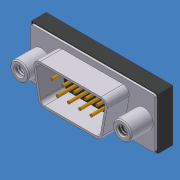
# Autodesk Inventor part: cRIO-FRC 9M D-Shell
Saved by Autodesk Inventor 2011 (Build 150239000, 239)
## iProperties
Category: FRC Parts
Manager: Ed Sparks
Company: FirstCadLibrary
Shininess: 64.0
Length Units: 11269
Angle Units: 11279
Time Units: 11290
Mass Units: 11283
Length Display Precision: 3
Angle Display Precision: 2
Compacted: True
Part Number: cRIO-FRC 9M D-Shell
Document SubType Name: Modeling
Created: 2005-12-27
Material: ABS Plastic
Designer: Ed Sparks
Project: FIRST
Density: 1 g/cm^3
Density: 0.0
Volumn: 0.0
Area: 0.0
PropertySet Name: Model Information
Control State: 0
Master: False
Checked Out: False
Author: Ed Sparks
Keywords: FIRST
Autodesk Inventor part; units mm, degrees
ref_plane "YZ Plane" through (0, 0, 0) normal (1, 0, 0) x (0, 1, 0)
ref_plane "XZ Plane" through (0, 0, 0) normal (0, 1, 0) x (-1, 0, 0)
ref_plane "XY Plane" through (0, 0, 0) normal (0, 0, 1) x (1, 0, 0)
sketch "Sketch1" plane through (0, 0, 0) normal (0, 0, 1) x (1, 0, 0)
  line L0 (-15.405, 0) -> (15.405, 0)
  line L1 (15.405, 0) -> (15.405, 3.6)
  line L2 (15.405, 3.6) -> (8.48, 3.6)
  line L3 (8.48, 3.6) -> (8.48, 9.96)
  line L4 (8.48, 9.96) -> (-8.48, 9.96)
  line L5 (-8.48, 9.96) -> (-8.48, 3.6)
  line L6 (-8.48, 3.6) -> (-15.405, 3.6)
  line L7 (-15.405, 3.6) -> (-15.405, 0)
  point P0 (0, 0)
  point P1 (0, 0)
  dimension "d0" = 16.96
  dimension "d1" = 9.96
  dimension "d2" = 3.6
  dimension "d3" = 30.81
  constraints: 16 end point, 6 parallel, 3 equal length, 1 coincident, 1 horizontal, 1 midpoint, 1 perpendicular, 1 other
  measures "d0" distance of L3.end L4.end
  measures "d1" distance between parallel lines of L0 L4
  measures "d2" distance of L0.end L1.end
  measures "d3" distance of L0.start L0.end
extrude "Extrusion1" add sketch "Sketch1" along normal blind 0.0001
sketch "Sketch2" plane through (0, 0, 0) normal (0, 0, -1) x (-1, 0, 0)
  line L0 (15.405, 3.6) -> (15.405, 0) projected
  line L1 (-15.405, 0) -> (15.405, 0)
  line L2 (15.405, 0) -> (15.405, 12.58)
  line L3 (15.405, 12.58) -> (-15.405, 12.58)
  line L4 (-15.405, 12.58) -> (-15.405, 0)
  dimension "d6" = 12.58
  constraints: 8 end point, 2 parallel, 1 collinear, 1 horizontal, 1 perpendicular
  measures "d6" distance of L3.end L1.start
extrude "Extrusion2" add sketch "Sketch2" along normal blind 3.6
sketch "Sketch5" plane through (0, 0, -3.6) normal (0, 0, -1) x (-1, 0, 0)
  line L0 (15.405, 0) -> (-15.405, 0) projected
  line L1 (-15.405, 12.58) -> (15.405, 12.58) projected
  line L2 (-7.4102, 10.415) -> (7.4102, 10.415)
  line L3 (8.395, 9.2414) -> (7.293, 2.9914)
  line L4 (6.3081, 2.165) -> (-6.3081, 2.165)
  line L5 (-7.293, 2.9914) -> (-8.395, 9.2414)
  arc A0 (-7.4102, 10.415) -> (-8.395, 9.2414) centre (-7.4102, 9.415) ccw
  arc A1 (8.395, 9.2414) -> (7.4102, 10.415) centre (7.4102, 9.415) ccw
  arc A2 (-7.293, 2.9914) -> (-6.3081, 2.165) centre (-6.3081, 3.165) ccw
  arc A3 (6.3081, 2.165) -> (7.293, 2.9914) centre (6.3081, 3.165) ccw
  line L6 (0, 12.58) -> (0, 0) construction
  line L7 (0, 10.415) -> (0, 12.58) construction
  line L8 (0, 0) -> (0, 2.165) construction
  arc A4 (-7.4102, 10.915) -> (-8.8874, 9.1545) centre (-7.4102, 9.415) ccw
  line L9 (-7.4102, 10.915) -> (7.4102, 10.915)
  arc A5 (8.8874, 9.1545) -> (7.4102, 10.915) centre (7.4102, 9.415) ccw
  line L10 (8.8874, 9.1545) -> (7.7854, 2.9045)
  arc A6 (6.3081, 1.665) -> (7.7854, 2.9045) centre (6.3081, 3.165) ccw
  line L11 (6.3081, 1.665) -> (-6.3081, 1.665)
  arc A7 (-7.7854, 2.9045) -> (-6.3081, 1.665) centre (-6.3081, 3.165) ccw
  line L12 (-7.7854, 2.9045) -> (-8.8874, 9.1545)
  dimension "d22" = 100
  dimension "d23" = 100
  dimension "d24" = 1
  dimension "d25" = 1
  dimension "d26" = 8.25
  dimension "d27" = 16.79
  dimension "d29" = 0.5
  constraints: 22 end point, 16 point on circle, 8 centre point, 8 tangent, 4 midpoint, 3 parallel, 2 collinear, 2 equal radius, 2 point on line, 7 other
  measures "d22" angle of L5 L4
  measures "d23" angle of L3 L4
  measures "d24" radius of A0
  measures "d25" radius of A2
  measures "d26" distance between parallel lines of L4 L2
  measures "d27" distance of L3.start L5.end
  measures "d29" distance between parallel lines of L11 L4
extrude "Extrusion3" add sketch "Sketch5" along normal blind 5.9
sketch "Sketch6" plane through (0, 0, -3.6) normal (0, 0, -1) x (-1, 0, 0)
  line L0 (-15.405, 0) -> (-15.405, 12.58) projected
  line L1 (15.405, 0) -> (-15.405, 0) projected
  line L2 (15.405, 12.58) -> (15.405, 0) projected
  line L3 (-15.405, 12.58) -> (15.405, 12.58) projected
  line L4 (-7.4102, 10.915) -> (7.4102, 10.915) projected
  arc A0 (8.8874, 9.1545) -> (7.4102, 10.915) centre (7.4102, 9.415) ccw projected
  line L5 (8.8874, 9.1545) -> (7.7854, 2.9045) projected
  arc A1 (6.3081, 1.665) -> (7.7854, 2.9045) centre (6.3081, 3.165) ccw projected
  line L6 (6.3081, 1.665) -> (-6.3081, 1.665) projected
  arc A2 (-7.7854, 2.9045) -> (-6.3081, 1.665) centre (-6.3081, 3.165) ccw projected
  line L7 (-7.7854, 2.9045) -> (-8.8874, 9.1545) projected
  arc A3 (-7.4102, 10.915) -> (-8.8874, 9.1545) centre (-7.4102, 9.415) ccw projected
  line L8 (-15.155, 11.83) -> (-15.155, 0.75)
  line L9 (-14.655, 0.25) -> (14.655, 0.25)
  line L10 (15.155, 0.75) -> (15.155, 11.83)
  line L11 (14.655, 12.33) -> (-14.655, 12.33)
  line L12 (-8.395, 9.2414) -> (-7.293, 2.9914) projected
  arc A4 (-7.293, 2.9914) -> (-6.3081, 2.165) centre (-6.3081, 3.165) ccw projected
  line L13 (-6.3081, 2.165) -> (6.3081, 2.165) projected
  arc A5 (-14.655, 12.33) -> (-15.155, 11.83) centre (-14.655, 11.83) ccw
  arc A6 (15.155, 11.83) -> (14.655, 12.33) centre (14.655, 11.83) ccw
  arc A7 (14.655, 0.25) -> (15.155, 0.75) centre (14.655, 0.75) ccw
  arc A8 (-15.155, 0.75) -> (-14.655, 0.25) centre (-14.655, 0.75) ccw
  dimension "d32" = 0.25
  dimension "d33" = 0.5
  constraints: 8 end point, 8 point on circle, 8 tangent, 4 centre point, 3 equal radius, 3 other
  measures "d32" distance between parallel lines of L8 L0
  measures "d33" radius of A5
extrude "Extrusion4" add sketch "Sketch6" along normal blind 0.5 contours A5 L11 A6 L10 A7 L9 A8 L8
sketch "Sketch7" plane through (0, 0, -4.1) normal (0, 0, -1) x (-1, 0, 0)
  line L0 (-14.655, 12.33) -> (14.655, 12.33) projected
  line L1 (14.655, 0.25) -> (-14.655, 0.25) projected
  circle A0 centre (12.495, 6.29) radius 2.25
  line L2 (12.495, 6.29) -> (12.495, 12.33)
  line L3 (12.495, 6.29) -> (12.495, 0.25)
  line L4 (15.405, 12.58) -> (15.405, 0) projected
  dimension "d36" = 4.5
  dimension "d37" = 2.91
  constraints: 4 end point, 2 perpendicular, 2 point on line, 1 centre point, 1 collinear
  measures "d36" diameter of A0
  measures "d37" distance from line of L4 L2.start
extrude "Extrusion5" add sketch "Sketch7" along normal blind 5.4
sketch "Sketch8" plane through (-12.495, 6.29, -9.5) normal (0, 0, -1) x (-1, 0, 0)
  circle A0 centre (0, 0) radius 2.25 projected
  constraints: 1 coincident
hole "Hole2" at (-12.495, 6.29, -9.5) direction (0, 0, 1) diameter 2.156 end through all thread size "4-40 UNC" class "2B" standard "ANSI Unified Screw Threads"
chamfer "Chamfer2" distance 0.25 angle 45 2 edges at (-10.245, 6.29, -9.5) (-12.495, 5.212, -9.5)
mirror "Mirror2" about plane through (0, 0, 0) normal (1, 0, 0) of "Extrusion5", "Hole2", "Chamfer2"
sketch "Sketch9" plane through (0, 0, -3.6) normal (0, 0, -1) x (-1, 0, 0)
  line L0 (7.4102, 10.415) -> (-7.4102, 10.415) projected
  line L1 (-6.3081, 2.165) -> (6.3081, 2.165) projected
  line L2 (0, 2.165) -> (0, 10.415) construction
  line L3 (-1.7032, 7.71) -> (6.4948, 7.71) construction
  line L4 (-1.5161, 4.87) -> (6.4574, 4.87) construction
  line L5 (-1.7032, 7.71) -> (-1.7032, 10.415) construction
  line L6 (-1.5161, 4.87) -> (-1.5161, 2.165) construction
  line L7 (-1.37, 8.1856) -> (-1.37, 4.0304) construction
  circle A0 centre (0, 7.71) radius 0.335
  circle A1 centre (-1.37, 4.87) radius 0.335
  circle A2 centre (2.74, 7.71) radius 0.335
  circle A3 centre (1.37, 4.87) radius 0.335
  circle A4 centre (5.48, 7.71) radius 0.335
  circle A5 centre (4.11, 4.87) radius 0.335
  dimension "d49" = 2.84
  dimension "d50" = 1.37
  dimension "d51" = 0.67
  dimension "d54" = 2.74
  constraints: 12 end point, 6 centre point, 6 point on line, 4 perpendicular, 3 equal radius, 2 midpoint, 2 parallel, 1 horizontal, 8 other
  measures "d49" distance between parallel lines of L4 L3
  measures "d50" distance between parallel lines of L2 L7
  measures "d51" diameter of A0
  measures "d54" distance of A0.centre A2.centre
extrude "Extrusion6" add sketch "Sketch9" along normal blind 5
mirror "Mirror3" about plane through (0, 0, 0) normal (1, 0, 0) of "Extrusion6"
body "Solid1"
